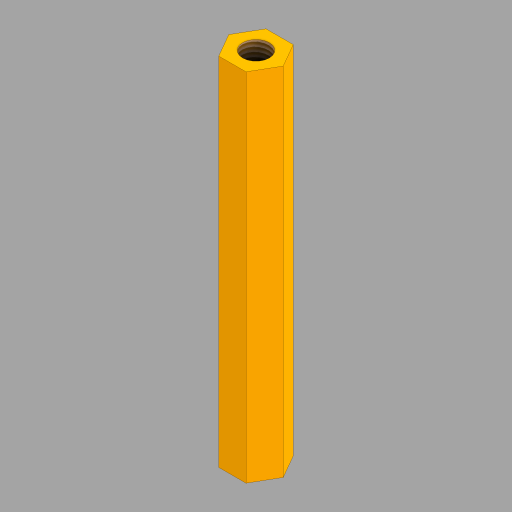
# Autodesk Inventor part: stoyka_M3_40mm
Saved by Autodesk Inventor 2024.2 (Build 282272000, 272)
## iProperties
Created: 2024-01-03
Part Number: stoyka_M3_40mm
Material: Типовые
Document SubType Name: Modeling
Designer: Fedor Orlov
Density: 1 g/cm^3
Appearance: По умолчанию
Author: Fedor Orlov
Autodesk Inventor part; units mm, degrees
ref_plane "YZ Plane" through (0, 0, 0) normal (1, 0, 0) x (0, 1, 0)
ref_plane "XZ Plane" through (0, 0, 0) normal (0, 1, 0) x (-1, 0, 0)
ref_plane "XY Plane" through (0, 0, 0) normal (0, 0, 1) x (1, 0, 0)
sketch "Эскиз1" plane through (0, 0, 0) normal (0, 1, 0) x (-1, 0, 0)
  line L0 (3.06, 0) -> (1.53, -2.65)
  line L1 (1.53, -2.65) -> (-1.53, -2.65)
  line L2 (-1.53, -2.65) -> (-3.06, 0)
  line L3 (-3.06, 0) -> (-1.53, 2.65)
  line L4 (-1.53, 2.65) -> (1.53, 2.65)
  line L5 (1.53, 2.65) -> (3.06, 0)
  circle A0 centre (0, 0) radius 1.5
  point P0 (0, -2.65)
  dimension "d0" = 5.3
  dimension "d1" = 5.3
  dimension "d2" = 3
  constraints: 12 end point, 2 coincident, 1 centre point, 1 midpoint, 13 other
  measures "d0" distance from line of point (0, -2.65) L4
  measures "d1" vertical distance of L0.end L3.end
  measures "d2" diameter of A0
extrude "Выдавливание1" add sketch "Эскиз1" along normal blind 40
thread "Резьба1" size "M3x0.5" class "6H" standard "ANSI Metric M Profile" full length
equation "\"d1\" = d0"
